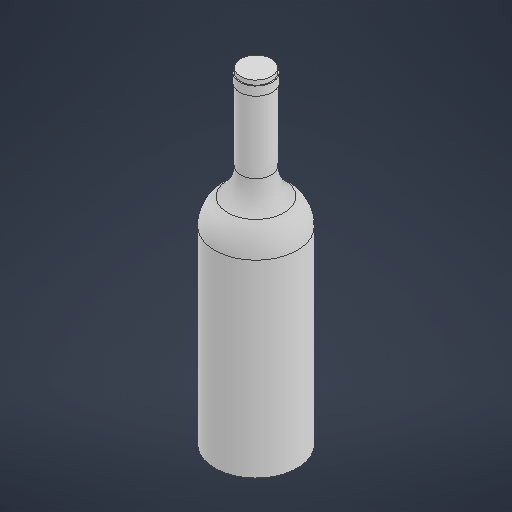
# Autodesk Inventor part: Botella_Vino
Saved by Autodesk Inventor 2026 (Build 300175050, 175E)
## iProperties
Created: 2025-12-08
Part Number: Botella_Vino
Material: Genérico
Document SubType Name: Modeling
Designer: David
Density: 1 g/cm^3
Appearance: Valor por defecto
Author: David
Autodesk Inventor part; units mm, degrees
ref_plane "YZ Plane" through (0, 0, 0) normal (1, 0, 0) x (0, 1, 0)
ref_plane "XZ Plane" through (0, 0, 0) normal (0, 1, 0) x (-1, 0, 0)
ref_plane "XY Plane" through (0, 0, 0) normal (0, 0, 1) x (1, 0, 0)
sketch "Boceto1" plane through (0, 0, 0) normal (0, 0, 1) x (1, 0, 0)
  point P0 (0, 0)
sketch "Boceto2" plane through (0, 0, 0) normal (0, 1, 0) x (-1, 0, 0)
  point P0 (0, 0)
sketch "Boceto3" plane through (0, 0, 0) normal (0, 1, 0) x (-1, 0, 0)
  circle A0 centre (0, 0) radius 37.5
  dimension "d0" = 75
  constraints: 1 centre point, 1 coincident
  measures "d0" diameter of A0
extrude "Extrusión1" add sketch "Boceto3" along normal blind 190
sketch "Boceto4" plane through (0, 190, 0) normal (0, 1, 0) x (1, 0, 0)
  circle A0 centre (0, 0) radius 14
  dimension "d3" = 28
  constraints: 1 centre point, 1 coincident
  measures "d3" diameter of A0
extrude "Extrusión2" add sketch "Boceto4" along normal blind 95
fillet "Empalme1" radius 30 1 edges at (-14, 190, 0)
fillet "Empalme2" radius 30 2 edges at (0, 190, -37.5) (0, 190, 37.5)
sketch "Boceto5" plane through (0, 285, 0) normal (0, 1, 0) x (1, 0, 0)
  circle A0 centre (0, 0) radius 15
  dimension "d8" = 30
  constraints: 1 centre point, 1 coincident
  measures "d8" diameter of A0
extrude "Extrusión3" add sketch "Boceto5" along normal blind 8
sketch "Boceto6" plane through (0, 293, 0) normal (0, 1, 0) x (1, 0, 0)
  circle A0 centre (0, 0) radius 14
  constraints: 1 centre point, 1 coincident
extrude "Extrusión4" add sketch "Boceto6" along normal blind 4
sketch "Boceto7" plane through (0, 0, 0) normal (0, -1, 0) x (1, 0, 0)
  circle A0 centre (0, 0) radius 2.5
  dimension "d13" = 5
  constraints: 1 centre point, 1 coincident
  measures "d13" diameter of A0
extrude "Extrusión5" cut sketch "Boceto7" against normal blind 18
fillet "Empalme3" radius 30 1 edges at (-2.5, 0, 0)
